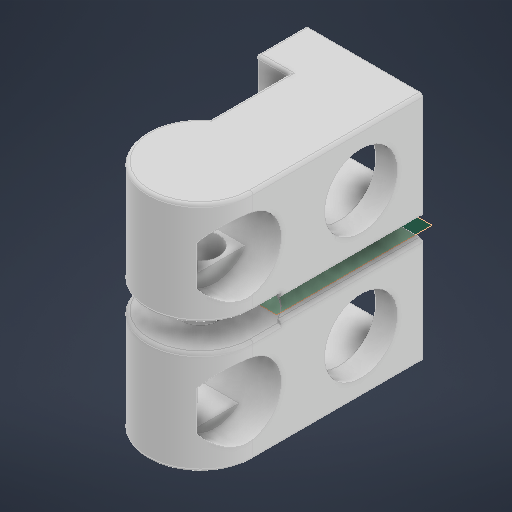
# Autodesk Inventor part: Lego leg
Saved by Autodesk Inventor 2027.1 (Build 311270010, 270A)
## iProperties
Created: 2020-11-13
Part Number: Lego leg
Material: Generic
Document SubType Name: Modeling
Designer: 164344
Density: 1 g/cm^3
Appearance: Default
Author: 164344
Autodesk Inventor part; units mm, degrees
ref_plane "YZ Plane" through (0, 0, 0) normal (1, 0, 0) x (0, 1, 0)
ref_plane "XZ Plane" through (0, 0, 0) normal (0, 1, 0) x (-1, 0, 0)
ref_plane "XY Plane" through (0, 0, 0) normal (0, 0, 1) x (1, 0, 0)
sketch "Sketch1" plane through (0, 0, 0) normal (0, 0, 1) x (1, 0, 0)
  line L0 (-3.91, -3.545) -> (3.91, -3.545)
  line L1 (3.91, -3.545) -> (3.91, 3.545)
  line L2 (3.91, 3.545) -> (-3.91, 3.545)
  line L3 (-3.91, 3.545) -> (-3.91, -3.545)
  line L4 (-3.91, -3.545) -> (3.91, 3.545) construction
  line L5 (3.91, -3.545) -> (-3.91, 3.545) construction
  point P0 (0, 0)
  dimension "d0" = 7.82
  dimension "d1" = 7.09
  constraints: 12 end point, 2 midpoint, 2 parallel, 1 horizontal, 1 perpendicular
  measures "d0" distance of L2.end L1.end
  measures "d1" distance of L1.end L0.end
extrude "Extrusion1" add sketch "Sketch1" along normal blind 3.26
sketch "Sketch2" plane through (0, 0, 3.26) normal (0, 0, 1) x (1, 0, 0)
  line L0 (3.91, 3.545) -> (-1.72, 3.545)
  line L1 (-1.72, 3.545) -> (-1.72, -3.545)
  line L2 (-1.72, -3.545) -> (3.91, -3.545)
  line L3 (3.91, -3.545) -> (3.91, 3.545)
  point P0 (0, 0)
  dimension "d5" = 5.63
  constraints: 8 end point, 2 parallel, 1 horizontal, 1 perpendicular
  measures "d5" distance of L0.start L0.end
extrude "Extrusion2" add sketch "Sketch2" along normal blind 8
sketch "Sketch3" plane through (-3.91, 3.545, 0) normal (0, 1, 0) x (1, 0, 0)
  line L0 (7.82, -11.26) -> (2.19, -11.26) projected
  circle A0 centre (4.32, -11.26) radius 3.5
  line L1 (7.82, 0) -> (7.82, -11.26) projected
  point P0 (3.91, 0)
  dimension "d10" = 7
  constraints: 1 centre point, 1 point on line, 1 tangent
  measures "d10" diameter of A0
extrude "Extrusion3" add sketch "Sketch3" against normal blind 7.09
sketch "Sketch4" plane through (0, 0, 0) normal (0, 0, -1) x (-1, 0, 0)
  line L0 (2.37, -2.545) -> (-2.47, -2.545)
  line L1 (-2.47, -2.545) -> (-2.47, 2.545)
  line L2 (-2.47, 2.545) -> (2.37, 2.545)
  line L3 (2.37, 2.545) -> (2.37, -2.545)
  line L4 (3.91, 3.545) -> (3.91, -3.545) projected
  line L5 (3.91, -3.545) -> (-3.91, -3.545) projected
  line L6 (-3.91, 3.545) -> (3.91, 3.545) projected
  line L7 (-3.91, -3.545) -> (-3.91, 3.545) projected
  point P0 (0, 0)
  dimension "d13" = 1.54
  dimension "d14" = 1
  dimension "d15" = 1
  dimension "d16" = 1.44
  constraints: 8 end point, 2 parallel, 1 horizontal, 1 perpendicular
  measures "d13" distance between parallel lines of L4 L3
  measures "d14" distance between parallel lines of L5 L0
  measures "d15" distance between parallel lines of L6 L2
  measures "d16" distance between parallel lines of L7 L1
extrude "Extrusion4" cut sketch "Sketch4" against normal blind 2.11 contours L0 L1 L2 L3
sketch "Sketch5" plane through (0, 0, 0) normal (0, 0, -1) x (-1, 0, 0)
  line L0 (-2.47, -2.545) -> (-2.47, 2.545) projected
  line L1 (-2.47, 2.545) -> (2.37, 2.545) projected
  line L2 (-2.47, -2.545) -> (0.88, -2.545)
  line L3 (0.88, -2.545) -> (0.88, 2.545)
  line L4 (0.88, 2.545) -> (-2.47, 2.545)
  line L5 (-2.47, 2.545) -> (-2.47, -2.545)
  point P0 (0, 0)
  dimension "d19" = 3.35
  constraints: 8 end point, 2 parallel, 1 horizontal, 1 perpendicular, 1 point on line
  measures "d19" distance between parallel lines of L3 L0
extrude "Extrusion5" cut sketch "Sketch5" against normal blind 7.2
sketch "Sketch6" plane through (3.91, -3.545, 0) normal (1, 0, 0) x (0, 0, -1)
  circle A0 centre (-4.08, 3.545) radius 2.435
  line L0 (0, 0) -> (0, 7.09) projected
  line L1 (0, 7.09) -> (-11.26, 7.09) projected
  point P0 (0, 3.545)
  dimension "d22" = 4.87
  dimension "d23" = 4.08
  dimension "d24" = 3.545
  constraints: 1 centre point
  measures "d22" diameter of A0
  measures "d23" distance from line of L0 A0.centre
  measures "d24" distance from line of L1 A0.centre
extrude "Extrusion6" cut sketch "Sketch6" against normal blind 2
sketch "Sketch7" plane through (3.91, -3.545, 0) normal (1, 0, 0) x (0, 0, -1)
  arc A0 (-13.8458, 2.24) -> (-13.8458, 4.85) centre (-11.79, 3.545) ccw
  line L0 (0, 0) -> (0, 7.09) projected
  line L1 (-13.8458, 2.24) -> (-13.8458, 4.85)
  line L2 (-14.76, 0) -> (-8.4828, 0) projected
  point P0 (0, 3.545)
  point P1 (-11.26, 0)
  dimension "d27" = 4.87
  dimension "d28" = 11.79
  dimension "d29" = 2.61
  dimension "d30" = 3.545
  constraints: 2 end point, 2 point on circle, 1 centre point, 1 vertical
  measures "d27" diameter of A0
  measures "d28" distance from line of L0 A0.centre
  measures "d29" distance of L1.end L1.start
  measures "d30" distance from line of A0.centre L2
extrude "Extrusion7" cut sketch "Sketch7" against normal blind 2
sketch "Sketch8" plane through (-3.91, -3.545, 0) normal (0, -1, 0) x (1, 0, 0)
  arc A0 (7.82, 11.26) -> (2.19, 8.4828) centre (4.32, 11.26) ccw projected
  circle A1 centre (4.32, 11.26) radius 3.8
  point P0 (3.91, 0)
  dimension "d33" = 7.6
  constraints: 1 centre point, 1 coincident
  measures "d33" diameter of A1
extrude "Extrusion8" cut sketch "Sketch8" against normal blind 0.23
sketch "Sketch9" plane through (-3.91, -3.315, 0) normal (0, -1, 0) x (1, 0, 0)
  arc A0 (7.82, 11.26) -> (2.19, 8.4828) centre (4.32, 11.26) ccw projected
  circle A1 centre (4.32, 11.26) radius 1.225
  point P0 (3.91, 0)
  dimension "d36" = 2.45
  constraints: 1 centre point, 1 coincident
  measures "d36" diameter of A1
extrude "Extrusion9" cut sketch "Sketch9" against normal blind 5
sketch "Sketch10" plane through (1.91, -3.545, 0) normal (1, 0, 0) x (0, 0, -1)
  arc A0 (-11.26, 1.1684) -> (-11.26, 5.9216) centre (-11.79, 3.545) ccw projected
  line L0 (-9.7406, 2.23) -> (-12.9615, 2.23)
  line L1 (-12.9615, 2.23) -> (-12.9857, 5.37)
  arc A1 (-9.7406, 2.23) -> (-10.178, 5.37) centre (-11.79, 3.545) ccw
  line L2 (-13.8458, 2.24) -> (-13.8458, 4.85) projected
  line L3 (-8.4828, 0.23) -> (-14.76, 0.23) projected
  line L4 (-8.4828, 7.09) -> (-14.76, 7.09) projected
  line L5 (-12.9857, 5.37) -> (-10.178, 5.37)
  line L6 (-10.035, 0.23) -> (-10.035, 5.23) projected
  line L7 (0, 7.09) -> (-11.26, 7.09) projected
  point P0 (0, 3.545)
  point P1 (-11.26, 0.23)
  dimension "d39" = 0.443
  dimension "d40" = 2
  dimension "d43" = 1.72
  constraints: 6 end point, 4 point on circle, 1 centre point, 1 horizontal, 1 perpendicular
  measures "d39" angle of L1 L2
  measures "d40" distance between parallel lines of L3 L0
  measures "d43" distance between parallel lines of L7 L5
extrude "Extrusion10" cut sketch "Sketch10" against normal blind 4 contours L0 L1 L5 A0
chamfer "Chamfer1" distance 0.4 angle 45 1 edges at (3.91, -3.43, 9.7801)
fillet "Fillet1" radius 0.2 12 edges at (3.91, 3.545, 5.63) (-1.1384, 3.545, 14.3989) (-1.72, 3.545, 5.8714) (-2.815, 3.545, 3.26) (-3.91, 0, 3.26) (-3.91, 3.545, 1.63) (-2.815, -3.545, 3.26) (3.91, -3.315, 10.5201) (-1.1384, -3.315, 14.3989) (-1.72, -3.545, 5.6865) (3.91, -3.545, 4.6901) (-3.91, -3.545, 1.63)
ref_plane "Work Plane1" through (-3.71, -4.175, 0) normal (0, -1, 0) x (1, 0, 0)
mirror "Mirror1" about plane through (-3.71, -4.175, 0) normal (0, -1, 0) of "Extrusion3", "Extrusion1", "Extrusion4", "Extrusion6", "Extrusion2", "Fillet1", "Extrusion5", "Extrusion10", "Extrusion7", "Extrusion9", "Extrusion8", "Chamfer1"
body "Solid1"
